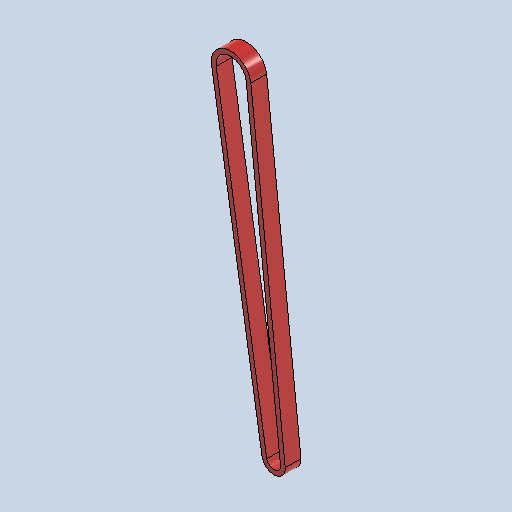
# Autodesk Inventor part: Angle Changer right band
Saved by Autodesk Inventor 2023.2 (Build 272271030, 271C)
## iProperties
Created: 2023-04-07
Part Number: Angle Changer right band
Material: Generic
Document SubType Name: Modeling
Designer: Main Account
Density: 1 g/cm^3
Appearance: Default
Author: Main Account
Autodesk Inventor part; units mm, degrees
ref_plane "YZ Plane" through (0, 0, 0) normal (1, 0, 0) x (0, 1, 0)
ref_plane "XZ Plane" through (0, 0, 0) normal (0, 1, 0) x (-1, 0, 0)
ref_plane "XY Plane" through (0, 0, 0) normal (0, 0, 1) x (1, 0, 0)
sketch "Sketch1" plane through (0, 0, 0) normal (0, 0, 1) x (1, 0, 0)
  circle A0 centre (0, 0) radius 4.7625 construction
  circle A1 centre (8.9141, -104.6721) radius 2.1844 construction
  arc A2 (6.7428, -104.9108) -> (11.0946, -104.5402) centre (8.9141, -104.6721) ccw
  arc A3 (4.7538, 0.2875) -> (-4.734, -0.5205) centre (0, 0) ccw
  line L0 (-4.734, -0.5205) -> (6.7428, -104.9108)
  line L1 (11.0946, -104.5402) -> (4.7538, 0.2875)
  line L2 (5.2518, -105.0747) -> (-6.225, -0.6844)
  arc A4 (6.2511, 0.3781) -> (-6.225, -0.6844) centre (0, 0) ccw
  line L3 (6.2511, 0.3781) -> (12.5918, -104.4496)
  arc A5 (5.2518, -105.0747) -> (12.5918, -104.4496) centre (8.9141, -104.6721) ccw
  point P0 (0, 0)
  dimension "d0" = 4.3688
  dimension "d1" = 1.5
  constraints: 8 end point, 8 point on circle, 4 centre point, 4 tangent, 2 coincident, 1 concentric, 3 other
  measures "d0" diameter of A2
  measures "d1" distance between parallel lines of L0 L2
extrude "Extrusion1" add sketch "Sketch1" along normal blind 5 and the other way blind 5
sketch "Sketch2" plane through (5.2518, -105.0747, -5) normal (-0.9940107, -0.1092827, 0) x (0, 0, 1)
  line L0 (0, 111.2818) -> (10, 111.2818) projected
  line L1 (10, 105.0193) -> (10, 0) projected
  line L2 (0, 0) -> (0, 105.0193) projected
  line L3 (0, -3.6844) -> (10, -3.6844) projected
  line L4 (0, 0) -> (0, -3.6844) projected
  line L5 (0, 0) -> (0, -3.6844)
  line L6 (10, -3.6844) -> (10, 0) projected
  line L7 (10, -3.6844) -> (10, 0)
  line L8 (10, 111.2818) -> (10, 105.0193)
  line L9 (10, 104.712) -> (10, 111.2818) projected
  line L10 (0, 111.2818) -> (0, 105.0193)
  line L11 (0, 111.2818) -> (0, 104.712) projected
  line L12 (5, -3.6844) -> (10, 111.2818)
  line L13 (0, -3.6844) -> (5, 111.2818)
  point P0 (5, 105.0193)
  point P1 (0, -0.1808)
  point P2 (10, -0.1808)
  dimension "d6" = 5
  dimension "d7" = 5
  constraints: 12 end point, 3 collinear, 2 midpoint, 1 vertical
  measures "d6" distance of L3.end L12.start
  measures "d7" distance of L0.start L13.end
extrude "Extrusion2" cut sketch "Sketch2" against normal blind 25.4 contours L0 L13 L4 L2 L10 | L8 L1 L6 L3 L12
body "Solid1"
